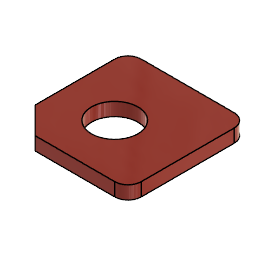
assambly of differrent parts (Autodesk Fusion 360 archive; units mm, degrees)
design "base_plate"
part number: 2026-08-04-15-53-25-718
Autodesk Fusion 360 part; units mm, degrees
sketch "Sketch1" plane through (0, 0, 0) normal (0, 0, 1) x (1, 0, 0)
  line L0 (0, 0) -> (80, 0)
  line L1 (90, 10) -> (90, 80)
  line L2 (80, 90) -> (10, 90)
  line L3 (0, 80) -> (0, 0)
  arc A0 (10, 90) -> (0, 80) centre (10, 80) ccw
  arc A1 (90, 80) -> (80, 90) centre (80, 80) ccw
  arc A2 (80, 0) -> (90, 10) centre (80, 10) ccw
  line L4 (0, 20) -> (20, 0)
  circle A3 centre (40, 40) radius 17.5
  point P0 (0, 90)
  dimension "d1" = 90
  dimension "d2" = 90
  dimension "d3" = 10
  dimension "d4" = 10
  dimension "d5" = 10
  dimension "d6" = 20
  dimension "d7" = 20
  dimension "d8" = 35
  dimension "d9" = 40
  dimension "d10" = 40
  constraint horizontal L0
  constraint vertical L1
  constraint horizontal L2
  constraint vertical L3
  constraint coincident L0.start L3.end
  constraint coincident P0 L3
  constraint coincident P0 L2
  constraint tangent L3 A0
  constraint tangent L2 A0
  constraint tangent L2 A1
  constraint tangent L1 A1
  constraint tangent L1 A2
  constraint tangent L0 A2
  constraint coincident L3 L4.start
  constraint coincident L0 L4.end
  measures "d1" distance of L0.start P0
  measures "d2" distance of L1 L3
  measures "d3" radius of A0
  measures "d4" radius of A1
  measures "d5" radius of A2
  measures "d6" distance of L0.start L4.start
  measures "d7" distance of L0.start L4.end
  measures "d8" diameter of A3
  measures "d9" distance of L3 A3.centre
  measures "d10" distance of L0 A3.centre
extrude "Extrude1" add sketch "Sketch1" along normal blind 10 contours L0 L1 L2 L3 A0 A1 A2 L4

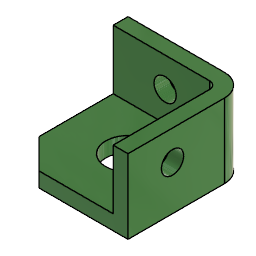
design "plate1"
part number: 2026-08-05-15-44-41-623
Autodesk Fusion 360 part; units mm, degrees
sketch "Sketch1" plane through (0, 0, 0) normal (0, 0, 1) x (1, 0, 0)
  line L0 (0, 0) -> (80, 0)
  line L1 (80, 0) -> (80, 80)
  line L2 (80, 80) -> (0, 80)
  line L3 (0, 80) -> (0, 0)
  circle A0 centre (40, 40) radius 15
  line L4 (0, 20) -> (20, 0)
  dimension "d1" = 80
  dimension "d2" = 80
  dimension "d3" = 30
  dimension "d4" = 40
  dimension "d5" = 40
  dimension "d6" = 20
  dimension "d7" = 20
  constraint horizontal L0
  constraint vertical L1
  constraint horizontal L2
  constraint vertical L3
  constraint coincident L0.start L3.end
  constraint coincident L3 L4.start
  constraint coincident L0 L4.end
  measures "d1" distance of L0.start L0.end
  measures "d2" distance of L0.start L2.end
  measures "d3" diameter of A0
  measures "d4" distance of L3 A0.centre
  measures "d5" distance of L0 A0.centre
  measures "d6" distance of L0.start L4.start
  measures "d7" distance of L0.start L4.end
extrude "Extrude1" add sketch "Sketch1" along normal blind 10 contours L0 L1 L2 L3 L4
sketch "Sketch2" plane through (0, 0, 10) normal (0, 0, 1) x (-1, 0, 0)
  circle A0 centre (-40, -40) radius 15
  line L0 (0, -20) -> (-20, 0)
  line L1 (-20, 0) -> (-80, 0)
  line L2 (-80, 0) -> (-80, -80)
  line L3 (-80, -80) -> (0, -80)
  line L4 (0, -80) -> (0, -20)
  line L5 (0, -80) -> (-80, -80)
  line L6 (-80, -80) -> (-80, -70)
  line L7 (-80, -70) -> (0, -70)
  line L8 (0, -70) -> (0, -80)
  line L9 (-80, -80) -> (-70, -80)
  line L10 (-70, -80) -> (-70, 0)
  line L11 (-70, 0) -> (-80, 0)
  line L12 (-80, 0) -> (-80, -80)
  dimension "d10" = 10
  dimension "d11" = 10
  constraint horizontal L5
  constraint vertical L6
  constraint horizontal L7
  constraint vertical L8
  constraint coincident L2 L6.end
  constraint coincident L3.end L4.start
  constraint horizontal L9
  constraint vertical L10
  constraint horizontal L11
  constraint vertical L12
  constraint coincident L1 L10.end
  constraint coincident L2.end L3.start
  measures "d10" distance of L3.end L7.end
  measures "d11" distance of L1.end L10.end
extrude "Extrude2" add sketch "Sketch2" along normal blind 40 contours L3 L4 L5 L7 L8 L10 | L1 L2 L7 L10 L11 L12 | L2 L3 L5 L6 L7 L9 L10 L12
fillet "Fillet1" radius 5 1 edges at (70, 70, 30)
fillet "Fillet2" radius 15 1 edges at (80, 80, 25)
sketch "Sketch3" plane through (70, 0, 0) normal (-1, 0, 0) x (0, -1, 0)
  line L0 (-65, 50) -> (-65, 10)
  line L1 (-65, 10) -> (0, 10)
  line L2 (0, 10) -> (0, 50)
  line L3 (0, 50) -> (-65, 50)
  circle A0 centre (-30, 30) radius 7.5
  dimension "d18" = 15
  dimension "d19" = 35
  dimension "d20" = 20
  measures "d18" diameter of A0
  measures "d19" distance of L0 A0.centre
  measures "d20" distance of L1 A0.centre
sketch "Sketch4" plane through (0, 70, 0) normal (0, -1, 0) x (1, 0, 0)
  line L0 (65, 10) -> (65, 50)
  line L1 (65, 50) -> (0, 50)
  line L2 (0, 50) -> (0, 10)
  line L3 (0, 10) -> (65, 10)
  circle A0 centre (35, 30) radius 7.5
  dimension "d21" = 15
  dimension "d22" = 35
  dimension "d23" = 20
  measures "d21" diameter of A0
  measures "d22" distance of L2 A0.centre
  measures "d23" distance of L3 A0.centre
extrude "Extrude3" cut sketch "Sketch4" against normal blind 10 contours A0
extrude "Extrude4" cut sketch "Sketch3" against normal blind 10 contours A0
